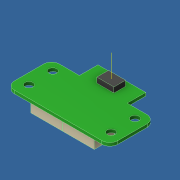
# Autodesk Inventor part: encoderR1_mini
Saved by Autodesk Inventor 2016 (Build 200138000, 138)
## iProperties
Created: 2016-03-31
Part Number: encoderR1_mini
Material: Generisch
Document SubType Name: Modeling
Designer: 4ndreas
Density: 1 g/cm^3
Appearance: Glatt - waldgrün
Mass: 1.82875 g
Surface Area: 21.1413 cm^2
Volume: 1.82875 cm^3
Author: 4ndreas
Autodesk Inventor part; units mm, degrees
ref_plane "YZ Plane" through (0, 0, 0) normal (1, 0, 0) x (0, 1, 0)
ref_plane "XZ Plane" through (0, 0, 0) normal (0, 1, 0) x (-1, 0, 0)
ref_plane "XY Plane" through (0, 0, 0) normal (0, 0, 1) x (1, 0, 0)
sketch "Skizze1" plane through (0, 0, 0) normal (0, 0, 1) x (1, 0, 0)
  line L0 (-19.5, -8.5) -> (19.5, -8.5)
  line L1 (19.5, -8.5) -> (19.5, 8.5)
  line L2 (19.5, 8.5) -> (-19.5, 8.5)
  line L3 (-19.5, 8.5) -> (-19.5, -8.5)
  line L4 (-19.5, -8.5) -> (19.5, 8.5) construction
  line L5 (19.5, -8.5) -> (-19.5, 8.5) construction
  line L6 (-9, 8.5) -> (9, 8.5)
  line L7 (9, 8.5) -> (9, 15.5)
  line L8 (9, 15.5) -> (-9, 15.5)
  line L9 (-9, 15.5) -> (-9, 8.5)
  line L10 (0, 15.5) -> (0, 0) construction
  line L11 (-15.5, -4) -> (15.5, -4) construction
  line L12 (15.5, -4) -> (15.5, 5) construction
  line L13 (15.5, 5) -> (-15.5, 5) construction
  line L14 (-15.5, 5) -> (-15.5, -4) construction
  line L15 (-3.233, 9.2988) -> (3.233, 9.2988)
  line L16 (3.233, 9.2988) -> (3.233, 13.7012)
  line L17 (3.233, 13.7012) -> (-3.233, 13.7012)
  line L18 (-3.233, 13.7012) -> (-3.233, 9.2988)
  line L19 (-3.233, 9.2988) -> (3.233, 13.7012) construction
  line L20 (3.233, 9.2988) -> (-3.233, 13.7012) construction
  line L21 (-15.5, -4) -> (15.5, -4)
  point P0 (0, 11.5)
  point P1 (0, -4)
  point P2 (0, 11.5)
  dimension "d0" = 39
  dimension "d2" = 24
  dimension "d3" = 7
  dimension "d5" = 20
  dimension "d8" = 4.5
  dimension "d9" = 13.5
  dimension "d23" = 31
  dimension "d24" = 15.5
  dimension "d25" = 9
  dimension "d37" = 31
  constraints: 44 end point, 8 parallel, 7 midpoint, 6 perpendicular, 4 horizontal, 3 point on line, 2 coincident, 2 other
  measures "d0" distance between parallel lines of L1 L3
  measures "d2" distance between parallel lines of L8 L0
  measures "d3" distance between parallel lines of L2 L8
  measures "d5" distance from line of point (0, 11.5) L0
  measures "d8" distance from line of L11.start L0
  measures "d9" distance from line of point (-15.5, 5) L0
  measures "d23" distance of L21.start L21.end
  measures "d24" distance from line of point (0, 11.5) L21
  measures "d25" distance between parallel lines of L9 L10
  measures "d37" distance between parallel lines of L14 L12
extrude "Extrusion1" add sketch "Skizze1" against normal blind 1.2 contours L3 L2 L1 L0 | L9 L8 L7 L2 | L18 L17 L16 L15
hole "Bohrung1" at (-15.5, 5, 0) at (-15.5, -4, 0) at (15.5, -4, 0) at (15.5, 5, 0) direction (0, 0, -1) diameter 3 end through all
extrude "Extrusion2" add sketch "Skizze1" along normal blind 2 contours L18 L17 L16 L15
sketch "Skizze2" plane through (0, 0, -1.2) normal (0, 0, -1) x (-1, 0, 0)
  circle A0 centre (-16.171, -4.461) radius 1.6729
  circle A1 centre (16.171, 5.5762) radius 1.6729
  circle A2 centre (16.171, -4.461) radius 1.6729
  circle A3 centre (-16.171, 5.5762) radius 1.6729
  line L0 (9, 8.5) -> (9, 15.5)
  line L1 (9, 15.5) -> (-9, 15.5)
  line L2 (-9, 15.5) -> (-9, 8.5)
  line L3 (-9, 8.5) -> (-19, 8.5)
  line L4 (-19, 8.5) -> (-19, -8.5)
  line L5 (-19, -8.5) -> (19, -8.5)
  line L6 (19, -8.5) -> (19, 8.5)
  line L7 (19, 8.5) -> (9, 8.5)
  line L8 (-11.95, -4.15) -> (-0.05, -4.15)
  line L9 (-0.05, -4.15) -> (-0.05, -11.75)
  line L10 (-0.05, -11.75) -> (-11.95, -11.75)
  line L11 (-11.95, -11.75) -> (-11.95, -4.15)
  line L12 (0.05, -4.15) -> (11.95, -4.15)
  line L13 (11.95, -4.15) -> (11.95, -11.75)
  line L14 (11.95, -11.75) -> (0.05, -11.75)
  line L15 (0.05, -11.75) -> (0.05, -4.15)
  line L16 (0, -0.9796) -> (0, 15.5) construction
  line L17 (-3.233, 9.2988) -> (-3.233, 13.7012)
  line L18 (-3.233, 13.7012) -> (3.233, 13.7012)
  line L19 (3.233, 13.7012) -> (3.233, 9.2988)
  line L20 (3.233, 9.2988) -> (-3.233, 9.2988)
  circle A4 centre (14.5, -4) radius 1.5
  circle A5 centre (-14.5, 5) radius 1.5
  circle A6 centre (-14.5, -4) radius 1.5
  circle A7 centre (14.5, 5) radius 1.5
  line L21 (9, 8.5) -> (9, 15.5)
  line L22 (9, 15.5) -> (-9, 15.5)
  line L23 (-9, 15.5) -> (-9, 8.5)
  line L24 (-9, 8.5) -> (-19, 8.5)
  line L25 (-19, 8.5) -> (-19, -8.5)
  line L26 (-19, -8.5) -> (19, -8.5)
  line L27 (19, -8.5) -> (19, 8.5)
  line L28 (19, 8.5) -> (9, 8.5)
  line L29 (9, 8.5) -> (9, 15.5)
  line L30 (-9, 15.5) -> (-9, 8.5)
  line L31 (-12.6037, -5.5) -> (13.7273, -5.5)
  line L32 (-19, -8.5) -> (19, -8.5)
  dimension "d26" = 11.9
  dimension "d27" = 0.1
  dimension "d28" = 7.6
  dimension "d29" = 3
  dimension "d30" = 6.25
  constraints: 66 end point, 8 centre point, 7 collinear, 4 parallel, 3 horizontal, 2 perpendicular, 1 midpoint, 1 point on line, 4 other
  measures "d26" distance between parallel lines of L11 L9
  measures "d27" distance between parallel lines of L15 L9
  measures "d28" distance between parallel lines of L14 L12
  measures "d29" distance between parallel lines of L26 L31
  measures "d30" distance between parallel lines of L31 L14
extrude "Extrusion3" [suppressed]
sketch "Skizze3" plane through (0, 0, -1.2) normal (0, 0, -1) x (-1, 0, 0)
  line L0 (12.6037, -5.5) -> (-13.7273, -5.5)
  line L1 (-11.95, -6.85) -> (-0.05, -6.85)
  line L2 (-0.05, -6.85) -> (-0.05, 0.75)
  line L3 (-0.05, 0.75) -> (-11.95, 0.75)
  line L4 (-11.95, 0.75) -> (-11.95, -6.85)
  line L5 (0.05, 0.75) -> (11.95, 0.75)
  line L6 (11.95, 0.75) -> (11.95, -6.85)
  line L7 (11.95, -6.85) -> (0.05, -6.85)
  line L8 (0.05, -6.85) -> (0.05, 0.75)
  line L9 (0, 0) -> (0, 11.5)
  dimension "d31" = 11.9
  dimension "d32" = 7.6
  dimension "d33" = 6.25
  dimension "d34" = 0.1
  constraints: 20 end point, 4 parallel, 2 equal length, 2 horizontal, 2 perpendicular, 1 vertical, 2 other
  measures "d31" distance between parallel lines of L4 L2
  measures "d32" distance between parallel lines of L3 L1
  measures "d33" distance between parallel lines of L0 L3
  measures "d34" distance between parallel lines of L2 L8
extrude "Extrusion4" add sketch "Skizze3" along normal blind 4.8
fillet "Rundung1" radius 3 4 edges at (-19.5, -8.5, -0.6) (-19.5, 8.5, -0.6) (19.5, -8.5, -0.6) (19.5, 8.5, -0.6)
equation "\"d24\" = 0.5 * d23"
equation "\"d37\" = d23"
equation "\"d31\" = d26"
equation "\"d32\" = d28"
equation "\"d33\" = d30"
equation "\"d34\" = d27"
